Autodesk Fusion 360 part; units mm, degrees
(part 2 of 3)
  line L468 (-37.8496, 96.7032) -> (-37.9919, 96.7743)
  line L469 (-37.9919, 96.7743) -> (-38.4187, 97.2011)
  line L470 (-38.4187, 97.2011) -> (-38.7032, 97.45)
  line L471 (-38.7032, 97.45) -> (-38.7743, 97.5923)
  line L472 (-38.7743, 97.5923) -> (-38.632, 97.9835)
  line L473 (-38.632, 97.9835) -> (-38.632, 98.3747)
  line L474 (-38.632, 98.3747) -> (-38.7387, 98.6948)
  line L475 (-38.7387, 98.6948) -> (-39.0588, 99.0504)
  line L476 (-39.0588, 99.0504) -> (-39.45, 99.1927)
  line L477 (-39.45, 99.1927) -> (-39.8412, 99.1927)
  line L478 (-39.8412, 99.1927) -> (-40.2324, 99.0504)
  line L479 (-40.2324, 99.0504) -> (-40.4458, 98.8726)
  line L480 (-40.4458, 98.8726) -> (-40.6236, 98.5881)
  line L481 (-40.6236, 98.5881) -> (-40.6948, 98.3036)
  line L482 (-40.6948, 98.3036) -> (-40.6948, 98.019)
  line L483 (-40.6948, 98.019) -> (-40.5525, 97.6278)
  line L484 (-40.5525, 97.6278) -> (-40.3036, 97.3433)
  line L485 (-40.3036, 97.3433) -> (-40.019, 97.2011)
  line L486 (-40.019, 97.2011) -> (-39.7345, 97.1299)
  line L487 (-39.7345, 97.1299) -> (-39.3078, 97.1299)
  line L488 (-39.3078, 97.1299) -> (-39.0588, 96.881)
  line L489 (-39.0588, 96.881) -> (-38.7743, 96.632)
  line L490 (-38.7743, 96.632) -> (-38.4898, 96.3475)
  line L491 (-38.4898, 96.3475) -> (-38.5609, 96.2053)
  line L492 (-38.5609, 96.2053) -> (-38.9521, 95.8496)
  line L493 (-38.9521, 95.8496) -> (-39.2011, 95.5651)
  line L494 (-39.2011, 95.5651) -> (-39.3078, 95.5651)
  line L495 (-39.3078, 95.5651) -> (-39.699, 95.8852)
  line L496 (-39.699, 95.8852) -> (-40.1969, 96.312)
  line L497 (-40.1969, 96.312) -> (-40.3036, 96.3831)
  line L498 (-40.3036, 96.3831) -> (-41.7617, 96.4187)
  line L499 (-41.7617, 96.4187) -> (-42.1173, 96.7743)
  line L500 (-42.1173, 96.7743) -> (-42.4374, 96.9166)
  line L501 (-42.4374, 96.9166) -> (-42.5797, 96.9521)
  line L502 (-42.5797, 96.9521) -> (-43.042, 96.9521)
  line L503 (-43.042, 96.9521) -> (-43.4332, 96.8099)
  line L504 (-43.4332, 96.8099) -> (-43.7177, 96.5965)
  line L505 (-43.7177, 96.5965) -> (-43.9311, 96.2408)
  line L506 (-43.9311, 96.2408) -> (-44.0022, 95.9919)
  line L507 (-44.0022, 95.9919) -> (-44.0022, 95.5651)
  line L508 (-44.0022, 95.5651) -> (-43.86, 95.1739)
  line L509 (-43.86, 95.1739) -> (-43.5399, 94.8183)
  line L510 (-43.5399, 94.8183) -> (-43.291, 94.676)
  line L511 (-43.291, 94.676) -> (-43.0064, 94.6049)
  line L512 (-43.0064, 94.6049) -> (-42.6152, 94.6049)
  line L513 (-42.6152, 94.6049) -> (-42.2596, 94.7116)
  line L514 (-42.2596, 94.7116) -> (-41.9751, 94.925)
  line L515 (-41.9751, 94.925) -> (-41.7973, 95.1383)
  line L516 (-41.7973, 95.1383) -> (-41.655, 95.4584)
  line L517 (-41.655, 95.4584) -> (-41.5839, 95.7785)
  line L518 (-41.5839, 95.7785) -> (-40.5881, 95.7785)
  line L519 (-40.5881, 95.7785) -> (-40.1969, 95.4229)
  line L520 (-40.1969, 95.4229) -> (-39.8057, 95.1028)
  line L521 (-39.8057, 95.1028) -> (-39.6634, 94.925)
  line L522 (-39.6634, 94.925) -> (-40.019, 94.2848)
  line L523 (-40.019, 94.2848) -> (-40.2324, 93.7869)
  line L524 (-40.2324, 93.7869) -> (-40.268, 93.7513)
  line L525 (-40.268, 93.7513) -> (-44.6068, 93.7158)
  line L526 (-44.6068, 93.7158) -> (-44.7847, 93.538)
  line L527 (-44.7847, 93.538) -> (-44.7491, 93.2534)
  line L528 (-44.7491, 93.2534) -> (-44.6068, 93.1467)
  line L529 (-44.6068, 93.1467) -> (-40.7303, 93.1112)
  line L530 (-40.7303, 93.1112) -> (-40.4814, 93.0756)
  line L531 (-40.4814, 93.0756) -> (-40.5169, 92.72)
  line L532 (-40.5169, 92.72) -> (-40.5881, 92.1154)
  line L533 (-40.5881, 92.1154) -> (-40.6236, 92.0798)
  line L534 (-40.6236, 92.0798) -> (-45.816, 92.0798)
  line L535 (-45.816, 92.0798) -> (-45.816, 93.1112)
  line L536 (-45.816, 93.1112) -> (-45.6738, 94.2137)
  line L537 (-45.6738, 94.2137) -> (-45.4604, 95.1383)
  line L538 (-45.4604, 95.1383) -> (-45.2114, 95.8852)
  line L539 (-45.2114, 95.8852) -> (-44.9269, 96.5253)
  line L540 (-44.9269, 96.5253) -> (-44.5713, 97.1655)
  line L541 (-44.5713, 97.1655) -> (-44.1801, 97.699)
  line L542 (-44.1801, 97.699) -> (-43.86, 98.0902)
  line L543 (-43.86, 98.0902) -> (-43.6466, 98.3391)
  line L544 (-43.6466, 98.3391) -> (-43.3621, 98.5881)
  line L545 (-43.3621, 98.5881) -> (-42.8998, 98.9793)
  line L546 (-42.8998, 98.9793) -> (-42.1529, 99.4416)
  line L547 (-42.1529, 99.4416) -> (-41.5127, 99.7261)
  line L548 (-41.5127, 99.7261) -> (-40.837, 99.9395)
  line L549 (-40.837, 99.9395) -> (-40.3036, 100.0462)
  line L550 (-40.3036, 100.0462) -> (-39.9835, 100.0818)
  line L551 (-34.6488, 95.1739) -> (-34.0087, 95.1383)
  line L552 (-34.0087, 95.1383) -> (-33.333, 94.9605)
  line L553 (-33.333, 94.9605) -> (-32.7639, 94.676)
  line L554 (-32.7639, 94.676) -> (-32.3016, 94.3559)
  line L555 (-32.3016, 94.3559) -> (-31.8393, 93.8936)
  line L556 (-31.8393, 93.8936) -> (-31.5192, 93.4313)
  line L557 (-31.5192, 93.4313) -> (-31.2702, 92.8622)
  line L558 (-31.2702, 92.8622) -> (-31.128, 92.3288)
  line L559 (-31.128, 92.3288) -> (-31.0924, 92.0798)
  line L560 (-31.0924, 92.0798) -> (-31.0924, 91.4041)
  line L561 (-31.0924, 91.4041) -> (-31.1991, 90.7995)
  line L562 (-31.1991, 90.7995) -> (-31.4836, 90.0882)
  line L563 (-31.4836, 90.0882) -> (-31.8037, 89.6259)
  line L564 (-31.8037, 89.6259) -> (-32.3016, 89.128)
  line L565 (-32.3016, 89.128) -> (-32.6572, 88.879)
  line L566 (-32.6572, 88.879) -> (-33.2618, 88.559)
  line L567 (-33.2618, 88.559) -> (-33.7242, 88.4167)
  line L568 (-33.7242, 88.4167) -> (-34.1509, 88.3456)
  line L569 (-34.1509, 88.3456) -> (-35.0045, 88.3456)
  line L570 (-35.0045, 88.3456) -> (-35.6091, 88.4523)
  line L571 (-35.6091, 88.4523) -> (-36.107, 88.6301)
  line L572 (-36.107, 88.6301) -> (-36.6404, 88.9146)
  line L573 (-36.6404, 88.9146) -> (-36.9961, 89.1991)
  line L574 (-36.9961, 89.1991) -> (-37.3517, 89.5548)
  line L575 (-37.3517, 89.5548) -> (-37.6718, 90.0171)
  line L576 (-37.6718, 90.0171) -> (-37.9208, 90.515)
  line L577 (-37.9208, 90.515) -> (-38.063, 90.9773)
  line L578 (-38.063, 90.9773) -> (-38.1341, 91.4397)
  line L579 (-38.1341, 91.4397) -> (-38.1341, 92.0798)
  line L580 (-38.1341, 92.0798) -> (-37.9919, 92.6844)
  line L581 (-37.9919, 92.6844) -> (-37.8496, 93.0045)
  line L582 (-37.8496, 93.0045) -> (-37.7785, 93.0045)
  line L583 (-37.7785, 93.0045) -> (-37.7785, 91.4397)
  line L584 (-37.7785, 91.4397) -> (-37.6362, 90.8351)
  line L585 (-37.6362, 90.8351) -> (-37.3873, 90.266)
  line L586 (-37.3873, 90.266) -> (-37.0317, 89.7681)
  line L587 (-37.0317, 89.7681) -> (-36.7116, 89.4481)
  line L588 (-36.7116, 89.4481) -> (-36.3559, 89.1991)
  line L589 (-36.3559, 89.1991) -> (-35.7869, 88.9146)
  line L590 (-35.7869, 88.9146) -> (-35.3246, 88.7723)
  line L591 (-35.3246, 88.7723) -> (-35.1467, 88.7368)
  line L592 (-35.1467, 88.7368) -> (-34.0798, 88.7368)
  line L593 (-34.0798, 88.7368) -> (-33.5108, 88.879)
  line L594 (-33.5108, 88.879) -> (-33.0129, 89.0924)
  line L595 (-33.0129, 89.0924) -> (-32.515, 89.4481)
  line L596 (-32.515, 89.4481) -> (-32.1949, 89.7681)
  line L597 (-32.1949, 89.7681) -> (-31.9104, 90.1593)
  line L598 (-31.9104, 90.1593) -> (-31.6259, 90.7284)
  line L599 (-31.6259, 90.7284) -> (-31.4836, 91.3685)
  line L600 (-31.4836, 91.3685) -> (-31.4836, 92.1154)
  line L601 (-31.4836, 92.1154) -> (-31.6614, 92.7911)
  line L602 (-31.6614, 92.7911) -> (-31.8393, 93.2179)
  line L603 (-31.8393, 93.2179) -> (-32.1949, 93.7158)
  line L604 (-32.1949, 93.7158) -> (-32.6572, 94.1781)
  line L605 (-32.6572, 94.1781) -> (-33.1196, 94.4626)
  line L606 (-33.1196, 94.4626) -> (-33.5108, 94.6404)
  line L607 (-33.5108, 94.6404) -> (-34.0443, 94.7827)
  line L608 (-34.0443, 94.7827) -> (-34.0087, 94.7471)
  line L609 (-34.0087, 94.7471) -> (-33.4397, 94.4982)
  line L610 (-33.4397, 94.4982) -> (-32.9062, 94.1781)
  line L611 (-32.9062, 94.1781) -> (-32.4439, 93.7513)
  line L612 (-32.4439, 93.7513) -> (-32.1238, 93.3601)
  line L613 (-32.1238, 93.3601) -> (-31.8393, 92.7911)
  line L614 (-31.8393, 92.7911) -> (-31.697, 92.2932)
  line L615 (-31.697, 92.2932) -> (-31.6614, 92.0443)
  line L616 (-31.6614, 92.0443) -> (-31.6614, 91.4752)
  line L617 (-31.6614, 91.4752) -> (-31.7326, 91.0485)
  line L618 (-31.7326, 91.0485) -> (-31.9104, 90.5506)
  line L619 (-31.9104, 90.5506) -> (-32.1593, 90.1238)
  line L620 (-32.1593, 90.1238) -> (-32.6217, 89.6259)
  line L621 (-32.6217, 89.6259) -> (-33.084, 89.3058)
  line L622 (-33.084, 89.3058) -> (-33.6175, 89.0569)
  line L623 (-33.6175, 89.0569) -> (-34.0798, 88.9502)
  line L624 (-34.0798, 88.9502) -> (-34.3999, 88.9146)
  line L625 (-34.3999, 88.9146) -> (-34.8267, 88.9146)
  line L626 (-34.8267, 88.9146) -> (-35.3246, 88.9857)
  line L627 (-35.3246, 88.9857) -> (-35.9647, 89.1991)
  line L628 (-35.9647, 89.1991) -> (-36.3204, 89.4125)
  line L629 (-36.3204, 89.4125) -> (-36.676, 89.697)
  line L630 (-36.676, 89.697) -> (-36.9605, 89.9815)
  line L631 (-36.9605, 89.9815) -> (-37.2806, 90.4794)
  line L632 (-37.2806, 90.4794) -> (-37.494, 90.9773)
  line L633 (-37.494, 90.9773) -> (-37.6007, 91.4752)
  line L634 (-37.6007, 91.4752) -> (-37.6007, 91.7597)
  line L635 (-37.6007, 91.7597) -> (-36.7116, 91.8309)
  line L636 (-36.7116, 91.8309) -> (-36.2492, 91.9376)
  line L637 (-36.2492, 91.9376) -> (-35.6802, 92.2221)
  line L638 (-35.6802, 92.2221) -> (-35.3246, 92.5066)
  line L639 (-35.3246, 92.5066) -> (-34.9689, 92.9689)
  line L640 (-34.9689, 92.9689) -> (-34.6844, 93.538)
  line L641 (-34.6844, 93.538) -> (-34.5777, 94.0003)
  line L642 (-34.5777, 94.0003) -> (-34.5777, 94.7116)
  line L643 (-34.5777, 94.7116) -> (-34.6844, 95.1383)
  line L644 (-34.6844, 95.1383) -> (-34.6488, 95.1739)
  line L645 (-35.1823, 95.8141) -> (-34.0087, 95.8141)
  line L646 (-34.0087, 95.8141) -> (-33.3685, 95.6718)
  line L647 (-33.3685, 95.6718) -> (-32.7995, 95.4584)
  line L648 (-32.7995, 95.4584) -> (-32.3372, 95.2095)
  line L649 (-32.3372, 95.2095) -> (-31.9104, 94.8894)
  line L650 (-31.9104, 94.8894) -> (-31.4836, 94.4982)
  line L651 (-31.4836, 94.4982) -> (-31.1635, 94.107)
  line L652 (-31.1635, 94.107) -> (-30.879, 93.6446)
  line L653 (-30.879, 93.6446) -> (-30.6301, 93.0756)
  line L654 (-30.6301, 93.0756) -> (-30.4878, 92.5422)
  line L655 (-30.4878, 92.5422) -> (-30.4167, 92.0087)
  line L656 (-30.4167, 92.0087) -> (-30.4167, 91.3685)
  line L657 (-30.4167, 91.3685) -> (-30.5234, 90.7284)
  line L658 (-30.5234, 90.7284) -> (-30.7368, 90.0882)
  line L659 (-30.7368, 90.0882) -> (-31.0213, 89.5548)
  line L660 (-31.0213, 89.5548) -> (-31.3414, 89.128)
  line L661 (-31.3414, 89.128) -> (-31.6614, 88.7723)
  line L662 (-31.6614, 88.7723) -> (-32.0882, 88.4167)
  line L663 (-32.0882, 88.4167) -> (-32.5861, 88.0966)
  line L664 (-32.5861, 88.0966) -> (-33.2974, 87.8121)
  line L665 (-33.2974, 87.8121) -> (-34.0087, 87.6698)
  line L666 (-34.0087, 87.6698) -> (-35.1823, 87.6698)
  line L667 (-35.1823, 87.6698) -> (-35.7869, 87.7765)
  line L668 (-35.7869, 87.7765) -> (-36.4626, 88.0255)
  line L669 (-36.4626, 88.0255) -> (-36.9605, 88.31)
  line L670 (-36.9605, 88.31) -> (-37.4584, 88.7012)
  line L671 (-37.4584, 88.7012) -> (-37.8496, 89.0924)
  line L672 (-37.8496, 89.0924) -> (-38.1697, 89.5192)
  line L673 (-38.1697, 89.5192) -> (-38.4187, 89.946)
  line L674 (-38.4187, 89.946) -> (-38.6676, 90.6217)
  line L675 (-38.6676, 90.6217) -> (-38.7743, 91.084)
  line L676 (-38.7743, 91.084) -> (-38.8099, 91.3685)
  line L677 (-38.8099, 91.3685) -> (-38.8099, 92.0443)
  line L678 (-38.8099, 92.0443) -> (-38.7032, 92.72)
  line L679 (-38.7032, 92.72) -> (-38.5253, 93.2534)
  line L680 (-38.5253, 93.2534) -> (-38.1341, 94.0003)
  line L681 (-38.1341, 94.0003) -> (-37.8496, 94.3559)
  line L682 (-37.8496, 94.3559) -> (-37.4584, 94.7827)
  line L683 (-37.4584, 94.7827) -> (-36.9961, 95.1383)
  line L684 (-36.9961, 95.1383) -> (-36.4271, 95.4584)
  line L685 (-36.4271, 95.4584) -> (-35.858, 95.6718)
  line L686 (-35.858, 95.6718) -> (-35.4313, 95.7785)
  line L687 (-35.4313, 95.7785) -> (-35.1823, 95.8141)
  line L688 (-34.6488, 95.1739) -> (-34.6844, 95.1028)
  line L689 (-34.6844, 95.1028) -> (-34.5777, 94.7116)
  line L690 (-34.5777, 94.7116) -> (-34.5777, 94.0003)
  line L691 (-34.5777, 94.0003) -> (-34.6844, 93.538)
  line L692 (-34.6844, 93.538) -> (-34.9689, 92.9689)
  line L693 (-34.9689, 92.9689) -> (-35.2179, 92.6488)
  line L694 (-35.2179, 92.6488) -> (-35.3957, 92.471)
  line L695 (-35.3957, 92.471) -> (-35.6802, 92.2221)
  line L696 (-35.6802, 92.2221) -> (-36.2492, 91.9376)
  line L697 (-36.2492, 91.9376) -> (-36.7116, 91.8309)
  line L698 (-36.7116, 91.8309) -> (-37.6007, 91.7597)
  line L699 (-37.6007, 91.7597) -> (-37.6007, 91.4752)
  line L700 (-37.6007, 91.4752) -> (-37.4584, 90.8706)
  line L701 (-37.4584, 90.8706) -> (-37.1739, 90.3016)
  line L702 (-37.1739, 90.3016) -> (-36.8894, 89.9104)
  line L703 (-36.8894, 89.9104) -> (-36.5693, 89.5903)
  line L704 (-36.5693, 89.5903) -> (-36.2137, 89.3414)
  line L705 (-36.2137, 89.3414) -> (-35.7869, 89.128)
  line L706 (-35.7869, 89.128) -> (-35.3246, 88.9857)
  line L707 (-35.3246, 88.9857) -> (-34.8267, 88.9146)
  line L708 (-34.8267, 88.9146) -> (-34.3999, 88.9146)
  line L709 (-34.3999, 88.9146) -> (-33.902, 88.9857)
  line L710 (-33.902, 88.9857) -> (-33.4397, 89.128)
  line L711 (-33.4397, 89.128) -> (-32.9062, 89.4125)
  line L712 (-32.9062, 89.4125) -> (-32.515, 89.7326)
  line L713 (-32.515, 89.7326) -> (-32.1593, 90.1238)
  line L714 (-32.1593, 90.1238) -> (-31.9104, 90.5506)
  line L715 (-31.9104, 90.5506) -> (-31.7326, 91.0485)
  line L716 (-31.7326, 91.0485) -> (-31.6614, 91.4752)
  line L717 (-31.6614, 91.4752) -> (-31.6614, 92.0443)
  line L718 (-31.6614, 92.0443) -> (-31.7681, 92.5777)
  line L719 (-31.7681, 92.5777) -> (-31.9815, 93.1112)
  line L720 (-31.9815, 93.1112) -> (-32.2305, 93.5024)
  line L721 (-32.2305, 93.5024) -> (-32.6217, 93.9292)
  line L722 (-32.6217, 93.9292) -> (-33.0129, 94.2492)
  line L723 (-33.0129, 94.2492) -> (-33.5819, 94.5693)
  line L724 (-33.5819, 94.5693) -> (-34.0087, 94.7471)
  line L725 (-34.0087, 94.7471) -> (-33.8664, 94.7471)
  line L726 (-33.8664, 94.7471) -> (-33.333, 94.5693)
  line L727 (-33.333, 94.5693) -> (-32.7995, 94.2848)
  line L728 (-32.7995, 94.2848) -> (-32.3727, 93.8936)
  line L729 (-32.3727, 93.8936) -> (-32.1238, 93.6446)
  line L730 (-32.1238, 93.6446) -> (-31.8037, 93.1467)
  line L731 (-31.8037, 93.1467) -> (-31.5903, 92.5777)
  line L732 (-31.5903, 92.5777) -> (-31.4836, 92.1154)
  line L733 (-31.4836, 92.1154) -> (-31.4836, 91.3685)
  line L734 (-31.4836, 91.3685) -> (-31.6259, 90.7284)
  line L735 (-31.6259, 90.7284) -> (-31.9104, 90.1593)
  line L736 (-31.9104, 90.1593) -> (-32.1238, 89.8748)
  line L737 (-32.1238, 89.8748) -> (-32.4439, 89.5192)
  line L738 (-32.4439, 89.5192) -> (-32.8351, 89.1991)
  line L739 (-32.8351, 89.1991) -> (-33.4041, 88.9146)
  line L740 (-33.4041, 88.9146) -> (-33.8664, 88.7723)
  line L741 (-33.8664, 88.7723) -> (-34.0798, 88.7368)
  line L742 (-34.0798, 88.7368) -> (-35.1467, 88.7368)
  line L743 (-35.1467, 88.7368) -> (-35.6802, 88.879)
  line L744 (-35.6802, 88.879) -> (-36.107, 89.0569)
  line L745 (-36.107, 89.0569) -> (-36.4626, 89.2702)
  line L746 (-36.4626, 89.2702) -> (-36.8183, 89.5548)
  line L747 (-36.8183, 89.5548) -> (-37.0672, 89.8037)
  line L748 (-37.0672, 89.8037) -> (-37.4229, 90.3372)
  line L749 (-37.4229, 90.3372) -> (-37.6362, 90.8351)
  line L750 (-37.6362, 90.8351) -> (-37.7785, 91.4397)
  line L751 (-37.7785, 91.4397) -> (-37.7785, 93.0045)
  line L752 (-37.7785, 93.0045) -> (-37.8852, 92.9689)
  line L753 (-37.8852, 92.9689) -> (-38.063, 92.4355)
  line L754 (-38.063, 92.4355) -> (-38.1341, 91.9731)
  line L755 (-38.1341, 91.9731) -> (-38.1341, 91.4397)
  line L756 (-38.1341, 91.4397) -> (-38.0274, 90.8351)
  line L757 (-38.0274, 90.8351) -> (-37.8141, 90.266)
  line L758 (-37.8141, 90.266) -> (-37.494, 89.7326)
  line L759 (-37.494, 89.7326) -> (-37.0672, 89.2702)
  line L760 (-37.0672, 89.2702) -> (-36.7471, 88.9857)
  line L761 (-36.7471, 88.9857) -> (-36.2492, 88.7012)
  line L762 (-36.2492, 88.7012) -> (-35.858, 88.5234)
  line L763 (-35.858, 88.5234) -> (-35.289, 88.3811)
  line L764 (-35.289, 88.3811) -> (-35.0045, 88.3456)
  line L765 (-35.0045, 88.3456) -> (-34.1509, 88.3456)
  line L766 (-34.1509, 88.3456) -> (-33.5819, 88.4523)
  line L767 (-33.5819, 88.4523) -> (-33.1196, 88.6301)
  line L768 (-33.1196, 88.6301) -> (-32.5861, 88.9146)
  line L769 (-32.5861, 88.9146) -> (-32.1949, 89.2347)
  line L770 (-32.1949, 89.2347) -> (-31.7681, 89.6614)
  line L771 (-31.7681, 89.6614) -> (-31.4125, 90.2305)
  line L772 (-31.4125, 90.2305) -> (-31.1991, 90.7995)
  line L773 (-31.1991, 90.7995) -> (-31.0924, 91.4041)
  line L774 (-31.0924, 91.4041) -> (-31.0924, 92.0798)
  line L775 (-31.0924, 92.0798) -> (-31.1991, 92.6488)
  line L776 (-31.1991, 92.6488) -> (-31.4125, 93.2179)
  line L777 (-31.4125, 93.2179) -> (-31.6259, 93.6091)
  line L778 (-31.6259, 93.6091) -> (-31.946, 94.0003)
  line L779 (-31.946, 94.0003) -> (-32.3372, 94.3915)
  line L780 (-32.3372, 94.3915) -> (-32.8706, 94.7471)
  line L781 (-32.8706, 94.7471) -> (-33.4397, 94.9961)
  line L782 (-33.4397, 94.9961) -> (-34.0087, 95.1383)
  line L783 (-34.0087, 95.1383) -> (-34.6488, 95.1739)
  line L784 (-31.5548, 105.5231) -> (-31.4125, 105.4875)
  line L785 (-31.4125, 105.4875) -> (-30.7723, 104.8474)
  line L786 (-30.7723, 104.8474) -> (-30.8079, 104.7051)
  line L787 (-30.8079, 104.7051) -> (-31.4481, 104.065)
  line L788 (-31.4481, 104.065) -> (-31.7681, 103.6738)
  line L789 (-31.7681, 103.6738) -> (-32.1949, 103.1403)
  line L790 (-32.1949, 103.1403) -> (-32.6572, 102.429)
  line L791 (-32.6572, 102.429) -> (-32.9773, 101.8956)
  line L792 (-32.9773, 101.8956) -> (-33.333, 101.1487)
  line L793 (-33.333, 101.1487) -> (-33.653, 100.2596)
  line L794 (-33.653, 100.2596) -> (-33.8309, 99.3705)
  line L795 (-33.8309, 99.3705) -> (-34.2576, 99.2994)
  line L796 (-34.2576, 99.2994) -> (-34.8978, 99.2994)
  line L797 (-34.8978, 99.2994) -> (-35.289, 99.3705)
  line L798 (-35.289, 99.3705) -> (-35.4313, 99.9395)
  line L799 (-35.4313, 99.9395) -> (-35.6446, 100.3663)
  line L800 (-35.6446, 100.3663) -> (-35.858, 100.6152)
  line L801 (-35.858, 100.6152) -> (-36.0359, 100.6864)
  line L802 (-36.0359, 100.6864) -> (-36.7116, 100.6864)
  line L803 (-36.7116, 100.6864) -> (-37.3873, 100.7931)
  line L804 (-37.3873, 100.7931) -> (-37.9208, 100.9709)
  line L805 (-37.9208, 100.9709) -> (-38.5253, 101.2554)
  line L806 (-38.5253, 101.2554) -> (-38.9877, 101.5755)
  line L807 (-38.9877, 101.5755) -> (-39.3789, 101.8956)
  line L808 (-39.3789, 101.8956) -> (-39.7345, 102.2512)
  line L809 (-39.7345, 102.2512) -> (-40.0902, 102.7135)
  line L810 (-40.0902, 102.7135) -> (-40.4814, 103.3537)
  line L811 (-40.4814, 103.3537) -> (-40.7303, 103.8516)
  line L812 (-40.7303, 103.8516) -> (-40.9793, 104.5984)
  line L813 (-40.9793, 104.5984) -> (-41.0504, 104.8829)
  line L814 (-41.0504, 104.8829) -> (-41.0504, 105.0608)
  line L815 (-41.0504, 105.0608) -> (-40.9437, 105.0963)
  line L816 (-40.9437, 105.0963) -> (-40.4458, 105.1319)
  line L817 (-40.4458, 105.1319) -> (-39.699, 105.1319)
  line L818 (-39.699, 105.1319) -> (-38.881, 105.0252)
  line L819 (-38.881, 105.0252) -> (-38.1341, 104.8118)
  line L820 (-38.1341, 104.8118) -> (-37.6007, 104.5984)
  line L821 (-37.6007, 104.5984) -> (-37.1028, 104.3139)
  line L822 (-37.1028, 104.3139) -> (-36.6049, 103.9583)
  line L823 (-36.6049, 103.9583) -> (-36.2848, 103.6738)
  line L824 (-36.2848, 103.6738) -> (-36.0359, 103.3892)
  line L825 (-36.0359, 103.3892) -> (-35.7158, 102.9625)
  line L826 (-35.7158, 102.9625) -> (-35.4313, 102.429)
  line L827 (-35.4313, 102.429) -> (-35.2534, 101.8956)
  line L828 (-35.2534, 101.8956) -> (-35.1467, 101.291)
  line L829 (-35.1467, 101.291) -> (-34.8978, 100.9709)
  line L830 (-34.8978, 100.9709) -> (-34.6844, 100.5441)
  line L831 (-34.6844, 100.5441) -> (-34.6133, 100.3663)
  line L832 (-34.6133, 100.3663) -> (-34.2221, 101.5399)
  line L833 (-34.2221, 101.5399) -> (-33.8664, 102.3223)
  line L834 (-33.8664, 102.3223) -> (-33.4041, 103.1403)
  line L835 (-33.4041, 103.1403) -> (-32.9773, 103.7805)
  line L836 (-32.9773, 103.7805) -> (-32.5861, 104.3139)
  line L837 (-32.5861, 104.3139) -> (-32.0882, 104.9185)
  line L838 (-32.0882, 104.9185) -> (-31.7681, 105.2742)
  line L839 (-31.7681, 105.2742) -> (-31.5548, 105.5231)
  line L840 (-34.471, 79.3834) -> (-32.7284, 79.3834)
  line L841 (-32.7284, 79.3834) -> (-32.4439, 79.2767)
  line L842 (-32.4439, 79.2767) -> (-32.266, 79.1344)
  line L843 (-32.266, 79.1344) -> (-32.1593, 78.8855)
  line L844 (-32.1593, 78.8855) -> (-32.1593, 78.5298)
  line L845 (-32.1593, 78.5298) -> (-32.266, 78.3165)
  line L846 (-32.266, 78.3165) -> (-32.515, 78.1031)
  line L847 (-32.515, 78.1031) -> (-32.7995, 78.0319)
  line L848 (-32.7995, 78.0319) -> (-33.8664, 78.0319)
  line L849 (-33.8664, 78.0319) -> (-33.8309, 77.214)
  line L850 (-33.8309, 77.214) -> (-33.7953, 77.1073)
  line L851 (-33.7953, 77.1073) -> (-34.471, 77.1073)
  line L852 (-34.471, 77.1073) -> (-34.471, 77.1784)
  line L853 (-34.471, 77.1784) -> (-34.3999, 77.1784)
  line L854 (-34.3999, 77.1784) -> (-34.3999, 79.2767)
  line L855 (-34.3999, 79.2767) -> (-34.471, 79.3834)
  line L856 (-37.0672, 79.3834) -> (-35.3601, 79.3834)
  line L857 (-35.3601, 79.3834) -> (-35.0401, 79.2767)
  line L858 (-35.0401, 79.2767) -> (-34.8267, 79.0277)
  line L859 (-34.8267, 79.0277) -> (-34.7555, 78.7788)
  line L860 (-34.7555, 78.7788) -> (-34.7911, 78.4587)
  line L861 (-34.7911, 78.4587) -> (-35.0045, 78.1742)
  line L862 (-35.0045, 78.1742) -> (-35.2179, 78.0675)
  line L863 (-35.2179, 78.0675) -> (-35.4313, 78.0319)
  line L864 (-35.4313, 78.0319) -> (-36.4626, 77.9964)
  line L865 (-36.4626, 77.9964) -> (-36.4626, 77.3562)
  line L866 (-36.4626, 77.3562) -> (-36.3915, 77.1073)
  line L867 (-36.3915, 77.1073) -> (-37.0672, 77.1073)
  line L868 (-37.0672, 77.1073) -> (-36.9961, 77.4629)
  line L869 (-36.9961, 77.4629) -> (-36.9961, 79.3123)
  line L870 (-36.9961, 79.3123) -> (-37.0672, 79.3123)
  line L871 (-37.0672, 79.3123) -> (-37.0672, 79.3834)
  line L872 (-27.287, 79.4901) -> (-27.2515, 79.4901)
  line L873 (-27.2515, 79.4901) -> (-27.2515, 78.921)
  line L874 (-27.2515, 78.921) -> (-27.3226, 78.921)
  line L875 (-27.3226, 78.921) -> (-27.3226, 78.9922)
  line L876 (-27.3226, 78.9922) -> (-28.8163, 78.9922)
  line L877 (-28.8163, 78.9922) -> (-28.8163, 78.4943)
  line L878 (-28.8163, 78.4943) -> (-27.8205, 78.4943)
  line L879 (-27.8205, 78.4943) -> (-27.8205, 78.5654)
  line L880 (-27.8205, 78.5654) -> (-27.7494, 78.5654)
  line L881 (-27.7494, 78.5654) -> (-27.7494, 78.0319)
  line L882 (-27.7494, 78.0319) -> (-27.8561, 78.0675)
  line L883 (-27.8561, 78.0675) -> (-28.8519, 78.1031)
  line L884 (-28.8519, 78.1031) -> (-28.8519, 77.4985)
  line L885 (-28.8519, 77.4985) -> (-27.3226, 77.534)
  line L886 (-27.3226, 77.534) -> (-27.2159, 77.5696)
  line L887 (-27.2159, 77.5696) -> (-27.2159, 77.0361)
  line L888 (-27.2159, 77.0361) -> (-27.3226, 77.0717)
  line L889 (-27.3226, 77.0717) -> (-29.4209, 77.1073)
  line L890 (-29.4209, 77.1073) -> (-29.3853, 77.214)
  line L891 (-29.3853, 77.214) -> (-29.3853, 79.2767)
  line L892 (-29.3853, 79.2767) -> (-29.4209, 79.3834)
  line L893 (-29.4209, 79.3834) -> (-27.3582, 79.4189)
  line L894 (-27.3582, 79.4189) -> (-27.287, 79.4901)
  line L895 (-39.0944, 79.3834) -> (-38.312, 79.3834)
  line L896 (-38.312, 79.3834) -> (-38.3475, 79.17)
  line L897 (-38.3475, 79.17) -> (-37.9563, 78.352)
  line L898 (-37.9563, 78.352) -> (-37.4229, 77.2851)
  line L899 (-37.4229, 77.2851) -> (-37.2806, 77.1428)
  line L900 (-37.2806, 77.1428) -> (-37.3162, 77.1073)
  line L901 (-37.3162, 77.1073) -> (-38.0986, 77.1073)
  line L902 (-38.0986, 77.1073) -> (-38.0274, 77.2851)
  line L903 (-38.0274, 77.2851) -> (-38.1697, 77.6052)
  line L904 (-38.1697, 77.6052) -> (-38.1697, 77.6763)
  line L905 (-38.1697, 77.6763) -> (-39.0588, 77.6763)
  line L906 (-39.0588, 77.6763) -> (-39.2366, 77.6407)
  line L907 (-39.2366, 77.6407) -> (-39.3789, 77.3207)
  line L908 (-39.3789, 77.3207) -> (-39.3789, 77.214)
  line L909 (-39.3789, 77.214) -> (-39.3078, 77.1784)
  line L910 (-39.3078, 77.1784) -> (-39.3078, 77.1073)
  line L911 (-39.3078, 77.1073) -> (-40.019, 77.1073)
  line L912 (-40.019, 77.1073) -> (-40.0546, 77.1784)
  line L913 (-40.0546, 77.1784) -> (-39.8768, 77.3562)
  line L914 (-39.8768, 77.3562) -> (-39.5923, 77.9964)
  line L915 (-39.5923, 77.9964) -> (-39.3078, 78.5654)
  line L916 (-39.3078, 78.5654) -> (-39.0232, 79.17)
  line L917 (-39.0232, 79.17) -> (-39.0944, 79.3834)
  line L918 (-31.8393, 79.3834) -> (-31.1635, 79.3834)
  line L919 (-31.1635, 79.3834) -> (-31.2347, 79.2411)
  line L920 (-31.2347, 79.2411) -> (-31.2347, 77.534)
  line L921 (-31.2347, 77.534) -> (-29.7765, 77.534)
  line L922 (-29.7765, 77.534) -> (-29.6698, 77.5696)
  line L923 (-29.6698, 77.5696) -> (-29.6698, 77.0717)
  line L924 (-29.6698, 77.0717) -> (-29.7765, 77.0361)
  line L925 (-29.7765, 77.0361) -> (-29.7765, 77.1073)
  line L926 (-29.7765, 77.1073) -> (-31.8393, 77.1073)
  line L927 (-31.8393, 77.1073) -> (-31.8037, 77.214)
  line L928 (-31.8037, 77.214) -> (-31.7681, 79.3123)
  line L929 (-31.7681, 79.3123) -> (-31.8393, 79.3123)
  line L930 (-31.8393, 79.3123) -> (-31.8393, 79.3834)
  line L931 (-26.4335, 89.4125) -> (-26.1846, 89.4125)
  line L932 (-26.1846, 89.4125) -> (-25.9356, 89.3058)
  line L933 (-25.9356, 89.3058) -> (-25.7222, 89.0569)
  line L934 (-25.7222, 89.0569) -> (-25.6867, 88.9502)
  line L935 (-25.6867, 88.9502) -> (-25.6867, 88.5945)
  line L936 (-25.6867, 88.5945) -> (-25.7933, 88.3811)
  line L937 (-25.7933, 88.3811) -> (-26.0779, 88.1677)
  line L938 (-26.0779, 88.1677) -> (-26.1846, 88.1322)
  line L939 (-26.1846, 88.1322) -> (-26.5046, 88.1322)
  line L940 (-26.5046, 88.1322) -> (-26.7536, 88.2744)
  line L941 (-26.7536, 88.2744) -> (-26.8958, 88.4523)
  line L942 (-26.8958, 88.4523) -> (-26.967, 88.6656)
  line L943 (-26.967, 88.6656) -> (-26.9314, 89.0213)
  line L944 (-26.9314, 89.0213) -> (-26.7891, 89.2347)
  line L945 (-26.7891, 89.2347) -> (-26.5758, 89.3769)
  line L946 (-26.5758, 89.3769) -> (-26.4335, 89.4125)
  line L947 (-43.042, 89.4125) -> (-42.7219, 89.3769)
  line L948 (-42.7219, 89.3769) -> (-42.5085, 89.2347)
  line L949 (-42.5085, 89.2347) -> (-42.3663, 89.0569)
  line L950 (-42.3663, 89.0569) -> (-42.2952, 88.7368)
  line L951 (-42.2952, 88.7368) -> (-42.4019, 88.4167)
  line L952 (-42.4019, 88.4167) -> (-42.6508, 88.2033)
  line L953 (-42.6508, 88.2033) -> (-42.8286, 88.1322)
  line L954 (-42.8286, 88.1322) -> (-43.0776, 88.1322)
  line L955 (-43.0776, 88.1322) -> (-43.3621, 88.2744)
  line L956 (-43.3621, 88.2744) -> (-43.5399, 88.4878)
  line L957 (-43.5399, 88.4878) -> (-43.5755, 88.5945)
  line L958 (-43.5755, 88.5945) -> (-43.5755, 88.9857)
  line L959 (-43.5755, 88.9857) -> (-43.4332, 89.1991)
  line L960 (-43.4332, 89.1991) -> (-43.2554, 89.3414)
  line L961 (-43.2554, 89.3414) -> (-43.042, 89.4125)
  line L962 (-40.9793, 79.3834) -> (-40.268, 79.3834)
  line L963 (-40.268, 79.3834) -> (-40.3391, 79.2767)
  line L964 (-40.3391, 79.2767) -> (-40.3391, 77.214)
  line L965 (-40.3391, 77.214) -> (-40.3036, 77.1073)
  line L966 (-40.3036, 77.1073) -> (-40.9437, 77.1073)
  line L967 (-40.9437, 77.1073) -> (-40.9793, 77.1784)
  line L968 (-40.9793, 77.1784) -> (-40.9082, 77.214)
  line L969 (-40.9082, 77.214) -> (-40.9082, 79.2767)
  line L970 (-40.9082, 79.2767) -> (-40.9793, 79.3834)
  line L971 (-26.3979, 96.3831) -> (-26.0423, 96.312)
  line L972 (-26.0423, 96.312) -> (-25.8289, 96.1341)
  line L973 (-25.8289, 96.1341) -> (-25.7222, 95.8852)
  line L974 (-25.7222, 95.8852) -> (-25.7578, 95.5651)
  line L975 (-25.7578, 95.5651) -> (-26.0067, 95.2806)
  line L976 (-26.0067, 95.2806) -> (-26.2912, 95.1739)
  line L977 (-26.2912, 95.1739) -> (-26.5758, 95.2095)
  line L978 (-26.5758, 95.2095) -> (-26.7891, 95.3517)
  line L979 (-26.7891, 95.3517) -> (-26.9314, 95.5651)
  line L980 (-26.9314, 95.5651) -> (-26.967, 95.8496)
  line L981 (-26.967, 95.8496) -> (-26.8603, 96.1341)
  line L982 (-26.8603, 96.1341) -> (-26.6469, 96.312)
  line L983 (-26.6469, 96.312) -> (-26.3979, 96.3831)
  line L984 (-42.8642, 96.3831) -> (-42.5797, 96.3475)
  line L985 (-42.5797, 96.3475) -> (-42.3307, 96.1697)
  line L986 (-42.3307, 96.1697) -> (-42.224, 95.9563)
  line L987 (-42.224, 95.9563) -> (-42.224, 95.6007)
  line L988 (-42.224, 95.6007) -> (-42.3307, 95.4229)
  line L989 (-42.3307, 95.4229) -> (-42.5441, 95.245)
  line L990 (-42.5441, 95.245) -> (-42.7219, 95.1739)
  line L991 (-42.7219, 95.1739) -> (-43.042, 95.2095)
  line L992 (-43.042, 95.2095) -> (-43.2554, 95.3517)
  line L993 (-43.2554, 95.3517) -> (-43.3977, 95.6007)
  line L994 (-43.3977, 95.6007) -> (-43.3977, 95.9919)
  line L995 (-43.3977, 95.9919) -> (-43.2554, 96.2053)
  line L996 (-43.2554, 96.2053) -> (-43.042, 96.3475)
  line L997 (-43.042, 96.3475) -> (-42.8642, 96.3831)
  line L998 (-27.287, 79.4901) -> (-27.2515, 79.4901)
  line L999 (-27.2515, 79.4901) -> (-27.2515, 78.921)
  line L1000 (-27.2515, 78.921) -> (-27.3226, 78.921)
  line L1001 (-27.3226, 78.921) -> (-27.3226, 78.9922)
  line L1002 (-27.3226, 78.9922) -> (-28.8163, 78.9922)
  line L1003 (-28.8163, 78.9922) -> (-28.8163, 78.4943)
  line L1004 (-28.8163, 78.4943) -> (-27.8205, 78.4943)
  line L1005 (-27.8205, 78.4943) -> (-27.8205, 78.5654)
  line L1006 (-27.8205, 78.5654) -> (-27.7494, 78.5654)
  line L1007 (-27.7494, 78.5654) -> (-27.7494, 78.0319)
  line L1008 (-27.7494, 78.0319) -> (-27.8561, 78.0675)
  line L1009 (-27.8561, 78.0675) -> (-28.8519, 78.1031)
  line L1010 (-28.8519, 78.1031) -> (-28.8519, 77.4985)
  line L1011 (-28.8519, 77.4985) -> (-27.3226, 77.534)
  line L1012 (-27.3226, 77.534) -> (-27.2159, 77.5696)
  line L1013 (-27.2159, 77.5696) -> (-27.2159, 77.0361)
  line L1014 (-27.2159, 77.0361) -> (-27.3226, 77.0717)
  line L1015 (-27.3226, 77.0717) -> (-29.4209, 77.1073)
  line L1016 (-29.4209, 77.1073) -> (-29.3853, 77.214)
  line L1017 (-29.3853, 77.214) -> (-29.3853, 79.2767)
  line L1018 (-29.3853, 79.2767) -> (-29.4209, 79.3834)
  line L1019 (-29.4209, 79.3834) -> (-27.3582, 79.4189)
  line L1020 (-27.3582, 79.4189) -> (-27.287, 79.4901)
  line L1021 (-29.2786, 79.3478) -> (-29.2786, 77.2851)
  line L1022 (-29.2786, 77.2851) -> (-29.2786, 77.1784)
  line L1023 (-29.2786, 77.1784) -> (-27.287, 77.1428)
  line L1024 (-27.287, 77.1428) -> (-27.2515, 77.1784)
  line L1025 (-27.2515, 77.1784) -> (-27.2515, 77.4629)
  line L1026 (-27.2515, 77.4629) -> (-28.8874, 77.4629)
  line L1027 (-28.8874, 77.4629) -> (-28.8874, 78.1031)
  line L1028 (-28.8874, 78.1031) -> (-28.8163, 78.1386)
  line L1029 (-28.8163, 78.1386) -> (-27.8561, 78.1742)
  line L1030 (-27.8561, 78.1742) -> (-27.7849, 78.3165)
  line L1031 (-27.7849, 78.3165) -> (-27.8205, 78.4231)
  line L1032 (-27.8205, 78.4231) -> (-28.8519, 78.4587)
  line L1033 (-28.8519, 78.4587) -> (-28.8874, 78.8855)
  line L1034 (-28.8874, 78.8855) -> (-28.8519, 79.0277)
  line L1035 (-28.8519, 79.0277) -> (-27.287, 79.0277)
  line L1036 (-27.287, 79.0277) -> (-27.3226, 79.3478)
  line L1037 (-27.3226, 79.3478) -> (-29.2786, 79.3478)
  line L1038 (-36.4271, 79.0277) -> (-35.6091, 79.0277)
  line L1039 (-35.6091, 79.0277) -> (-35.3601, 78.9566)
  line L1040 (-35.3601, 78.9566) -> (-35.289, 78.8499)
  line L1041 (-35.289, 78.8499) -> (-35.289, 78.5654)
  line L1042 (-35.289, 78.5654) -> (-35.4668, 78.4231)
  line L1043 (-35.4668, 78.4231) -> (-36.4626, 78.4231)
  line L1044 (-36.4626, 78.4231) -> (-36.4982, 78.4587)
  line L1045 (-36.4982, 78.4587) -> (-36.4982, 78.8855)
  line L1046 (-36.4982, 78.8855) -> (-36.4271, 79.0277)
  line L1047 (-33.8309, 79.0277) -> (-32.9773, 79.0277)
  line L1048 (-32.9773, 79.0277) -> (-32.7639, 78.9566)
  line L1049 (-32.7639, 78.9566) -> (-32.6572, 78.7788)
  line L1050 (-32.6572, 78.7788) -> (-32.6928, 78.5298)
  line L1051 (-32.6928, 78.5298) -> (-32.8706, 78.4231)
  line L1052 (-32.8706, 78.4231) -> (-33.8664, 78.4231)
  line L1053 (-33.8664, 78.4231) -> (-33.8664, 78.9922)
  line L1054 (-33.8664, 78.9922) -> (-33.8309, 79.0277)
  line L1055 (-39.0588, 83.4377) -> (-38.7387, 83.4377)
  line L1056 (-38.7387, 83.4377) -> (-38.5253, 83.2599)
  line L1057 (-38.5253, 83.2599) -> (-38.4542, 83.0821)
  line L1058 (-38.4542, 83.0821) -> (-38.4898, 82.8331)
  line L1059 (-38.4898, 82.8331) -> (-38.6676, 82.6197)
  line L1060 (-38.6676, 82.6197) -> (-38.9521, 82.5486)
  line L1061 (-38.9521, 82.5486) -> (-39.2011, 82.6553)
  line L1062 (-39.2011, 82.6553) -> (-39.3078, 82.762)
  line L1063 (-39.3078, 82.762) -> (-39.3433, 82.8687)
  line L1064 (-39.3433, 82.8687) -> (-39.3433, 83.1532)
  line L1065 (-39.3433, 83.1532) -> (-39.2366, 83.331)
  line L1066 (-39.2366, 83.331) -> (-39.0588, 83.4377)
  line L1067 (-30.4523, 83.4377) -> (-30.1677, 83.4377)
  line L1068 (-30.1677, 83.4377) -> (-29.9544, 83.2954)
  line L1069 (-29.9544, 83.2954) -> (-29.8477, 83.0465)
  line L1070 (-29.8477, 83.0465) -> (-29.8832, 82.8331)
  line L1071 (-29.8832, 82.8331) -> (-30.0611, 82.6197)
  line L1072 (-30.0611, 82.6197) -> (-30.3811, 82.5486)
  line L1073 (-30.3811, 82.5486) -> (-30.5945, 82.6553)
  line L1074 (-30.5945, 82.6553) -> (-30.7368, 82.8331)
  line L1075 (-30.7368, 82.8331) -> (-30.7368, 83.1888)
  line L1076 (-30.7368, 83.1888) -> (-30.559, 83.3666)
  line L1077 (-30.559, 83.3666) -> (-30.4523, 83.4377)
  line L1078 (-39.8057, 98.5881) -> (-39.4856, 98.5881)
  line L1079 (-39.4856, 98.5881) -> (-39.3078, 98.4814)
  line L1080 (-39.3078, 98.4814) -> (-39.2011, 98.268)
  line L1081 (-39.2011, 98.268) -> (-39.2011, 98.0546)
  line L1082 (-39.2011, 98.0546) -> (-39.3433, 97.8412)
  line L1083 (-39.3433, 97.8412) -> (-39.5211, 97.7345)
  line L1084 (-39.5211, 97.7345) -> (-39.8412, 97.7345)
  line L1085 (-39.8412, 97.7345) -> (-40.019, 97.9124)
  line L1086 (-40.019, 97.9124) -> (-40.0902, 98.0546)
  line L1087 (-40.0902, 98.0546) -> (-40.0902, 98.3036)
  line L1088 (-40.0902, 98.3036) -> (-39.9479, 98.5169)
  line L1089 (-39.9479, 98.5169) -> (-39.8057, 98.5881)
  line L1090 (-29.7054, 98.5881) -> (-29.3498, 98.5881)
  line L1091 (-29.3498, 98.5881) -> (-29.172, 98.4458)
  line L1092 (-29.172, 98.4458) -> (-29.1008, 98.3036)
  line L1093 (-29.1008, 98.3036) -> (-29.1008, 98.0546)
  line L1094 (-29.1008, 98.0546) -> (-29.2075, 97.8768)
  line L1095 (-29.2075, 97.8768) -> (-29.3142, 97.7701)
  line L1096 (-29.3142, 97.7701) -> (-29.4209, 97.7345)
  line L1097 (-29.4209, 97.7345) -> (-29.6698, 97.7345)
  line L1098 (-29.6698, 97.7345) -> (-29.8477, 97.8412)
  line L1099 (-29.8477, 97.8412) -> (-29.9544, 97.9835)
  line L1100 (-29.9544, 97.9835) -> (-29.9899, 98.2324)
  line L1101 (-29.9899, 98.2324) -> (-29.8832, 98.4814)
  line L1102 (-29.8832, 98.4814) -> (-29.7054, 98.5881)
  line L1103 (-27.3226, 86.6029) -> (-27.0025, 86.6029)
  line L1104 (-27.0025, 86.6029) -> (-26.7891, 86.4251)
  line L1105 (-26.7891, 86.4251) -> (-26.7536, 86.354)
  line L1106 (-26.7536, 86.354) -> (-26.7536, 86.0339)
  line L1107 (-26.7536, 86.0339) -> (-26.9314, 85.8205)
  line L1108 (-26.9314, 85.8205) -> (-27.1092, 85.7494)
  line L1109 (-27.1092, 85.7494) -> (-27.3582, 85.7849)
  line L1110 (-27.3582, 85.7849) -> (-27.536, 85.9272)
  line L1111 (-27.536, 85.9272) -> (-27.6071, 86.0695)
  line L1112 (-27.6071, 86.0695) -> (-27.6071, 86.3184)
  line L1113 (-27.6071, 86.3184) -> (-27.4649, 86.5318)
  line L1114 (-27.4649, 86.5318) -> (-27.3226, 86.6029)
  line L1115 (-42.1529, 86.6029) -> (-41.8684, 86.6029)
  line L1116 (-41.8684, 86.6029) -> (-41.655, 86.4607)
  line L1117 (-41.655, 86.4607) -> (-41.5839, 86.2828)
  line L1118 (-41.5839, 86.2828) -> (-41.5839, 86.0695)
  line L1119 (-41.5839, 86.0695) -> (-41.7261, 85.8561)
  line L1120 (-41.7261, 85.8561) -> (-41.9395, 85.7494)
  line L1121 (-41.9395, 85.7494) -> (-42.224, 85.7849)
  line L1122 (-42.224, 85.7849) -> (-42.4019, 85.9628)
  line L1123 (-42.4019, 85.9628) -> (-42.4374, 86.0339)
  line L1124 (-42.4374, 86.0339) -> (-42.4374, 86.354)
  line L1125 (-42.4374, 86.354) -> (-42.2952, 86.5318)
  line L1126 (-42.2952, 86.5318) -> (-42.1529, 86.6029)
  line L1127 (-39.0944, 79.3834) -> (-38.312, 79.3834)
  line L1128 (-38.312, 79.3834) -> (-38.3475, 79.17)
  line L1129 (-38.3475, 79.17) -> (-37.9563, 78.352)
  line L1130 (-37.9563, 78.352) -> (-37.4229, 77.2851)
  line L1131 (-37.4229, 77.2851) -> (-37.2806, 77.1428)
  line L1132 (-37.2806, 77.1428) -> (-37.3162, 77.1073)
  line L1133 (-37.3162, 77.1073) -> (-38.0986, 77.1073)
  line L1134 (-38.0986, 77.1073) -> (-38.0274, 77.2851)
  line L1135 (-38.0274, 77.2851) -> (-38.1697, 77.6052)
  line L1136 (-38.1697, 77.6052) -> (-38.1697, 77.6763)
  line L1137 (-38.1697, 77.6763) -> (-39.0588, 77.6763)
  line L1138 (-39.0588, 77.6763) -> (-39.2366, 77.6407)
  line L1139 (-39.2366, 77.6407) -> (-39.3789, 77.3207)
  line L1140 (-39.3789, 77.3207) -> (-39.3789, 77.214)
  line L1141 (-39.3789, 77.214) -> (-39.3078, 77.1784)
  line L1142 (-39.3078, 77.1784) -> (-39.3078, 77.1073)
  line L1143 (-39.3078, 77.1073) -> (-40.019, 77.1073)
  line L1144 (-40.019, 77.1073) -> (-40.0546, 77.1784)
  line L1145 (-40.0546, 77.1784) -> (-39.8768, 77.3562)
  line L1146 (-39.8768, 77.3562) -> (-39.5923, 77.9964)
  line L1147 (-39.5923, 77.9964) -> (-39.3078, 78.5654)
  line L1148 (-39.3078, 78.5654) -> (-39.0232, 79.17)
  line L1149 (-39.0232, 79.17) -> (-39.0944, 79.3834)
  line L1150 (-38.9166, 79.3478) -> (-39.0588, 78.9566)
  line L1151 (-39.0588, 78.9566) -> (-39.2011, 78.6721)
  line L1152 (-39.2011, 78.6721) -> (-39.4856, 78.0675)
  line L1153 (-39.4856, 78.0675) -> (-39.4856, 77.9252)
  line L1154 (-39.4856, 77.9252) -> (-39.5567, 77.9252)
  line L1155 (-39.5567, 77.9252) -> (-39.5923, 77.7119)
  line L1156 (-39.5923, 77.7119) -> (-39.6634, 77.7119)
  line L1157 (-39.6634, 77.7119) -> (-39.8768, 77.2495)
  line L1158 (-39.8768, 77.2495) -> (-39.9124, 77.1784)
  line L1159 (-39.9124, 77.1784) -> (-39.699, 77.1428)
  line L1160 (-39.699, 77.1428) -> (-39.4856, 77.1428)
  line L1161 (-39.4856, 77.1428) -> (-39.45, 77.1784)
  line L1162 (-39.45, 77.1784) -> (-39.4145, 77.534)
  line L1163 (-39.4145, 77.534) -> (-39.3433, 77.534)
  line L1164 (-39.3433, 77.534) -> (-39.2722, 77.7474)
  line L1165 (-39.2722, 77.7474) -> (-38.2053, 77.7119)
  line L1166 (-38.2053, 77.7119) -> (-38.063, 77.6763)
  line L1167 (-38.063, 77.6763) -> (-38.0986, 77.5696)
  line L1168 (-38.0986, 77.5696) -> (-38.0274, 77.5696)
  line L1169 (-38.0274, 77.5696) -> (-37.9919, 77.214)
  line L1170 (-37.9919, 77.214) -> (-37.9919, 77.1784)
  line L1171 (-37.9919, 77.1784) -> (-37.5295, 77.1784)
  line L1172 (-37.5295, 77.1784) -> (-37.4584, 77.2495)
  line L1173 (-37.4584, 77.2495) -> (-37.5295, 77.3918)
  line L1174 (-37.5295, 77.3918) -> (-37.6007, 77.3918)
  line L1175 (-37.6007, 77.3918) -> (-37.6362, 77.6052)
  line L1176 (-37.6362, 77.6052) -> (-37.9563, 78.2098)
  line L1177 (-37.9563, 78.2098) -> (-38.3475, 79.0277)
  line L1178 (-38.3475, 79.0277) -> (-38.4187, 79.2411)
  line L1179 (-38.4187, 79.2411) -> (-38.4187, 79.3478)
  line L1180 (-38.4187, 79.3478) -> (-38.9166, 79.3478)
  line L1181 (-31.8393, 79.3834) -> (-31.1635, 79.3834)
  line L1182 (-31.1635, 79.3834) -> (-31.2347, 79.2411)
  line L1183 (-31.2347, 79.2411) -> (-31.2347, 77.534)
  line L1184 (-31.2347, 77.534) -> (-29.7765, 77.534)
  line L1185 (-29.7765, 77.534) -> (-29.6698, 77.5696)
  line L1186 (-29.6698, 77.5696) -> (-29.6698, 77.0717)
  line L1187 (-29.6698, 77.0717) -> (-29.7765, 77.0361)
  line L1188 (-29.7765, 77.0361) -> (-29.7765, 77.1073)
  line L1189 (-29.7765, 77.1073) -> (-31.8393, 77.1073)
  line L1190 (-31.8393, 77.1073) -> (-31.8037, 77.214)
  line L1191 (-31.8037, 77.214) -> (-31.7681, 79.3123)
  line L1192 (-31.7681, 79.3123) -> (-31.8393, 79.3123)
  line L1193 (-31.8393, 79.3123) -> (-31.8393, 79.3834)
  line L1194 (-31.7326, 79.3478) -> (-31.7326, 77.1784)
  line L1195 (-31.7326, 77.1784) -> (-31.6614, 77.1428)
  line L1196 (-31.6614, 77.1428) -> (-29.8477, 77.1784)
  line L1197 (-29.8477, 77.1784) -> (-29.741, 77.1428)
  line L1198 (-29.741, 77.1428) -> (-29.741, 77.4629)
  line L1199 (-29.741, 77.4629) -> (-31.3058, 77.4273)
  line L1200 (-31.3058, 77.4273) -> (-31.3058, 79.2767)
  line L1201 (-31.3058, 79.2767) -> (-31.3414, 79.3478)
  line L1202 (-31.3414, 79.3478) -> (-31.7326, 79.3478)
  line L1203 (-34.471, 79.3834) -> (-32.7284, 79.3834)
  line L1204 (-32.7284, 79.3834) -> (-32.4439, 79.2767)
  line L1205 (-32.4439, 79.2767) -> (-32.266, 79.1344)
  line L1206 (-32.266, 79.1344) -> (-32.1593, 78.8855)
  line L1207 (-32.1593, 78.8855) -> (-32.1593, 78.5298)
  line L1208 (-32.1593, 78.5298) -> (-32.266, 78.3165)
  line L1209 (-32.266, 78.3165) -> (-32.515, 78.1031)
  line L1210 (-32.515, 78.1031) -> (-32.7995, 78.0319)
  line L1211 (-32.7995, 78.0319) -> (-33.8664, 78.0319)
  line L1212 (-33.8664, 78.0319) -> (-33.8309, 77.214)
  line L1213 (-33.8309, 77.214) -> (-33.7953, 77.1073)
  line L1214 (-33.7953, 77.1073) -> (-34.471, 77.1073)
  line L1215 (-34.471, 77.1073) -> (-34.471, 77.1784)
  line L1216 (-34.471, 77.1784) -> (-34.3999, 77.1784)
  line L1217 (-34.3999, 77.1784) -> (-34.3999, 79.2767)
  line L1218 (-34.3999, 79.2767) -> (-34.471, 79.3834)
  line L1219 (-34.3288, 79.3478) -> (-34.3288, 77.1784)
  line L1220 (-34.3288, 77.1784) -> (-33.902, 77.1784)
  line L1221 (-33.902, 77.1784) -> (-33.902, 78.0675)
  line L1222 (-33.902, 78.0675) -> (-32.6572, 78.1031)
  line L1223 (-32.6572, 78.1031) -> (-32.4083, 78.2098)
  line L1224 (-32.4083, 78.2098) -> (-32.3727, 78.352)
  line L1225 (-32.3727, 78.352) -> (-32.3016, 78.352)
  line L1226 (-32.3016, 78.352) -> (-32.2305, 78.4943)
  line L1227 (-32.2305, 78.4943) -> (-32.1949, 78.7788)
  line L1228 (-32.1949, 78.7788) -> (-32.3016, 79.0633)
  line L1229 (-32.3016, 79.0633) -> (-32.4794, 79.2411)
  line L1230 (-32.4794, 79.2411) -> (-32.6217, 79.3123)
  line L1231 (-32.6217, 79.3123) -> (-32.8706, 79.3478)
  line L1232 (-32.8706, 79.3478) -> (-34.3288, 79.3478)
  line L1233 (-37.0672, 79.3834) -> (-35.3601, 79.3834)
  line L1234 (-35.3601, 79.3834) -> (-35.0401, 79.2767)
  line L1235 (-35.0401, 79.2767) -> (-34.8267, 79.0277)
  line L1236 (-34.8267, 79.0277) -> (-34.7555, 78.7788)
  line L1237 (-34.7555, 78.7788) -> (-34.7911, 78.4587)
  line L1238 (-34.7911, 78.4587) -> (-34.8978, 78.352)
  line L1239 (-34.8978, 78.352) -> (-34.8622, 78.5298)
  line L1240 (-34.8622, 78.5298) -> (-34.8622, 78.8855)
  line L1241 (-34.8622, 78.8855) -> (-35.0045, 79.0989)
  line L1242 (-35.0045, 79.0989) -> (-35.0045, 79.17)
  line L1243 (-35.0045, 79.17) -> (-35.0756, 79.17)
  line L1244 (-35.0756, 79.17) -> (-35.0756, 79.2411)
  line L1245 (-35.0756, 79.2411) -> (-35.4313, 79.3123)
  line L1246 (-35.4313, 79.3123) -> (-36.925, 79.3478)
  line L1247 (-36.925, 79.3478) -> (-36.925, 77.214)
  line L1248 (-36.925, 77.214) -> (-36.5338, 77.1784)
  line L1249 (-36.5338, 77.1784) -> (-36.5693, 78.0675)
  line L1250 (-36.5693, 78.0675) -> (-36.3204, 78.1386)
  line L1251 (-36.3204, 78.1386) -> (-35.289, 78.1386)
  line L1252 (-35.289, 78.1386) -> (-35.2179, 78.1742)
  line L1253 (-35.2179, 78.1742) -> (-35.1467, 78.1031)
  line L1254 (-35.1467, 78.1031) -> (-35.4313, 78.0319)
  line L1255 (-35.4313, 78.0319) -> (-36.4626, 77.9964)
  line L1256 (-36.4626, 77.9964) -> (-36.4626, 77.3562)
  line L1257 (-36.4626, 77.3562) -> (-36.3915, 77.1073)
  line L1258 (-36.3915, 77.1073) -> (-37.0672, 77.1073)
  line L1259 (-37.0672, 77.1073) -> (-36.9961, 77.4629)
  line L1260 (-36.9961, 77.4629) -> (-36.9961, 79.3123)
  line L1261 (-36.9961, 79.3123) -> (-37.0672, 79.3123)
  line L1262 (-37.0672, 79.3123) -> (-37.0672, 79.3834)
  line L1263 (-40.9793, 79.3834) -> (-40.268, 79.3834)
  line L1264 (-40.268, 79.3834) -> (-40.3391, 79.2767)
  line L1265 (-40.3391, 79.2767) -> (-40.3391, 77.214)
  line L1266 (-40.3391, 77.214) -> (-40.3036, 77.1073)
  line L1267 (-40.3036, 77.1073) -> (-40.9437, 77.1073)
  line L1268 (-40.9437, 77.1073) -> (-40.9793, 77.1784)
  line L1269 (-40.9793, 77.1784) -> (-40.9082, 77.214)
  line L1270 (-40.9082, 77.214) -> (-40.9082, 79.2767)
  line L1271 (-40.9082, 79.2767) -> (-40.9793, 79.3834)
  line L1272 (-40.8015, 79.3478) -> (-40.837, 79.3123)
  line L1273 (-40.837, 79.3123) -> (-40.837, 77.1784)
  line L1274 (-40.837, 77.1784) -> (-40.4103, 77.1784)
  line L1275 (-40.4103, 77.1784) -> (-40.4103, 79.3123)
  line L1276 (-40.4103, 79.3123) -> (-40.4458, 79.3478)
  line L1277 (-40.4458, 79.3478) -> (-40.8015, 79.3478)
  line L1278 (-38.7387, 78.7788) -> (-38.5965, 78.6365)
  line L1279 (-38.5965, 78.6365) -> (-38.3475, 78.0319)
  line L1280 (-38.3475, 78.0319) -> (-38.3831, 77.9964)
  line L1281 (-38.3831, 77.9964) -> (-39.0232, 77.9964)
  line L1282 (-39.0232, 77.9964) -> (-39.0588, 78.1031)
  line L1283 (-39.0588, 78.1031) -> (-38.7387, 78.7788)
  line L1284 (-33.902, 79.0633) -> (-32.8706, 79.0633)
  line L1285 (-32.8706, 79.0633) -> (-32.6928, 78.9922)
  line L1286 (-32.6928, 78.9922) -> (-32.6217, 78.8499)
  line L1287 (-32.6217, 78.8499) -> (-32.6217, 78.5654)
  line L1288 (-32.6217, 78.5654) -> (-32.6572, 78.4231)
  line L1289 (-32.6572, 78.4231) -> (-32.9773, 78.352)
  line L1290 (-32.9773, 78.352) -> (-33.8664, 78.352)
  line L1291 (-33.8664, 78.352) -> (-33.9376, 78.5298)
  line L1292 (-33.9376, 78.5298) -> (-33.9376, 78.9922)
  line L1293 (-33.9376, 78.9922) -> (-33.902, 79.0633)
  line L1294 (-33.8309, 79.0277) -> (-33.8664, 78.9922)
  line L1295 (-33.8664, 78.9922) -> (-33.8664, 78.4231)
  line L1296 (-33.8664, 78.4231) -> (-32.8706, 78.4231)
  line L1297 (-32.8706, 78.4231) -> (-32.6928, 78.5298)
  line L1298 (-32.6928, 78.5298) -> (-32.6572, 78.7788)
  line L1299 (-32.6572, 78.7788) -> (-32.7639, 78.9566)
  line L1300 (-32.7639, 78.9566) -> (-32.9773, 79.0277)
  line L1301 (-32.9773, 79.0277) -> (-33.8309, 79.0277)
  line L1302 (-36.5338, 79.0633) -> (-35.5024, 79.0633)
  line L1303 (-35.5024, 79.0633) -> (-35.289, 78.9566)
  line L1304 (-35.289, 78.9566) -> (-35.1823, 78.7432)
  line L1305 (-35.1823, 78.7432) -> (-35.2179, 78.5298)
  line L1306 (-35.2179, 78.5298) -> (-35.289, 78.5298)
  line L1307 (-35.289, 78.5298) -> (-35.289, 78.4231)
  line L1308 (-35.289, 78.4231) -> (-35.6091, 78.3876)
  line L1309 (-35.6091, 78.3876) -> (-35.6446, 78.3165)
  line L1310 (-35.6446, 78.3165) -> (-36.4982, 78.352)
  line L1311 (-36.4982, 78.352) -> (-36.5338, 78.3876)
  line L1312 (-36.5338, 78.3876) -> (-36.5338, 79.0633)
  line L1313 (-36.4271, 79.0277) -> (-36.4982, 78.8855)
  line L1314 (-36.4982, 78.8855) -> (-36.4982, 78.4587)
  line L1315 (-36.4982, 78.4587) -> (-36.4626, 78.4231)
  line L1316 (-36.4626, 78.4231) -> (-35.4668, 78.4231)
  line L1317 (-35.4668, 78.4231) -> (-35.289, 78.5654)
  line L1318 (-35.289, 78.5654) -> (-35.289, 78.8499)
  line L1319 (-35.289, 78.8499) -> (-35.4313, 78.9922)
  line L1320 (-35.4313, 78.9922) -> (-35.6091, 79.0277)
  line L1321 (-35.6091, 79.0277) -> (-36.4271, 79.0277)
  line L1322 (-38.7387, 78.8499) -> (-38.632, 78.8144)
  line L1323 (-38.632, 78.8144) -> (-38.312, 78.1031)
  line L1324 (-38.312, 78.1031) -> (-38.312, 77.9608)
  line L1325 (-38.312, 77.9608) -> (-39.1299, 77.9608)
  line L1326 (-39.1299, 77.9608) -> (-39.0944, 78.1742)
  line L1327 (-39.0944, 78.1742) -> (-38.7743, 78.8144)
  line L1328 (-38.7743, 78.8144) -> (-38.7387, 78.8499)
  line L1329 (-38.7387, 78.7788) -> (-39.0588, 78.1031)
  line L1330 (-39.0588, 78.1031) -> (-39.0232, 77.9964)
  line L1331 (-39.0232, 77.9964) -> (-38.3831, 77.9964)
  line L1332 (-38.3831, 77.9964) -> (-38.3475, 78.0675)
  line L1333 (-38.3475, 78.0675) -> (-38.5965, 78.6365)
  line L1334 (-38.5965, 78.6365) -> (-38.7387, 78.7788)